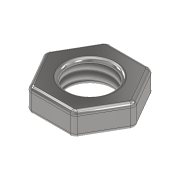
# Autodesk Inventor part: M2_nut
Saved by Autodesk Inventor 2020 (Build 240168000, 168)
## iProperties
Created: 2021-02-03
Part Number: M2_nut
Material: Generic
Document SubType Name: Modeling
Designer: JojoS
Density: 1 g/cm^3
Appearance: Steel - Polished
Author: JojoS
Autodesk Inventor part; units mm, degrees
ref_plane "YZ Plane" through (0, 0, 0) normal (1, 0, 0) x (0, 1, 0)
ref_plane "XZ Plane" through (0, 0, 0) normal (0, 1, 0) x (-1, 0, 0)
ref_plane "XY Plane" through (0, 0, 0) normal (0, 0, 1) x (1, 0, 0)
sketch "Sketch1" plane through (0, 0, 0) normal (0, 1, 0) x (-1, 0, 0)
  circle A0 centre (0, 0) radius 1.15
  line L0 (-1.1836, -2.05) -> (-2.3671, 0)
  line L1 (-2.3671, 0) -> (-1.1836, 2.05)
  line L2 (-1.1836, 2.05) -> (1.1836, 2.05)
  line L3 (1.1836, 2.05) -> (2.3671, 0)
  line L4 (2.3671, 0) -> (1.1836, -2.05)
  line L5 (1.1836, -2.05) -> (-1.1836, -2.05)
  dimension "d0" = 2.3
  dimension "d1" = 2.05
  constraints: 12 end point, 2 coincident, 1 centre point, 13 other
  measures "d0" diameter of A0
  measures "d1" distance from line of L5 point (0, 0)
extrude "Extrusion1" add sketch "Sketch1" along normal blind 1.2
fillet "Fillet1" radius 0.3 6 edges at (2.3671, 0.6, 0) (1.1836, 0.6, 2.05) (-1.1836, 0.6, 2.05) (-2.3671, 0.6, 0) (-1.1836, 0.6, -2.05) (1.1836, 0.6, -2.05)
thread "Thread1" size "M2.3x0.45" class "6H" standard "ANSI Metric M Profile" full length
fillet "Fillet2" radius 0.2 24 edges at (1.7754, 1.2, 1.025) (1.1604, 1.2, 2.0098) (0, 1.2, 2.05) (-1.1604, 1.2, 2.0098) (-1.7754, 1.2, 1.025) (-2.3207, 1.2, 0) (-1.7754, 1.2, -1.025) (-1.1604, 1.2, -2.0098) (0, 1.2, -2.05) (1.1604, 1.2, -2.0098) (1.7754, 1.2, -1.025) (2.3207, 1.2, 0) (1.7754, 0, -1.025) (1.1604, 0, -2.0098) (0, 0, -2.05) (-1.1604, 0, -2.0098) (-1.7754, 0, -1.025) (-2.3207, 0, 0) (-1.7754, 0, 1.025) (-1.1604, 0, 2.0098) (0, 0, 2.05) (1.1604, 0, 2.0098) (1.7754, 0, 1.025) (2.3207, 0, 0)
fillet "Fillet3" radius 0.2 2 edges at (1.15, 1.2, 0) (1.15, 0, 0)
body "Solid1"
